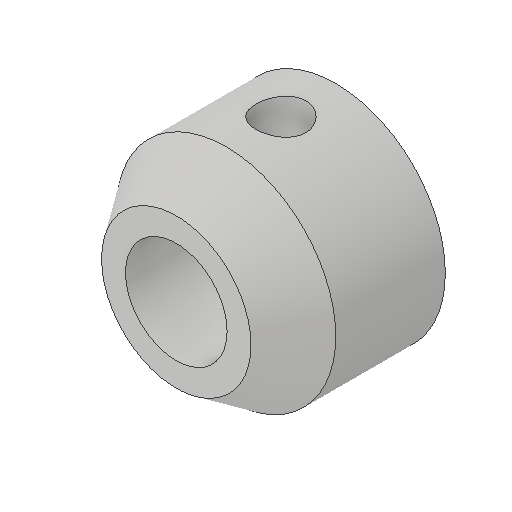
# Autodesk Inventor part: 3DP_PLA_X_axis_idler_shaft_locking_ring
Saved by Autodesk Inventor 2025 (Build 290162010, 162A)
## iProperties
Created: 2018-07-11
Part Number: 3DP_PLA_X_axis_idler_shaft_locking_ring
Material: Generic
Document SubType Name: Modeling
Designer: Andrzej
Density: 1 g/cm^3
Appearance: Default
Author: Andrzej
Autodesk Inventor part; units mm, degrees
ref_plane "YZ Plane" through (0, 0, 0) normal (1, 0, 0) x (0, 1, 0)
ref_plane "XZ Plane" through (0, 0, 0) normal (0, 1, 0) x (-1, 0, 0)
ref_plane "XY Plane" through (0, 0, 0) normal (0, 0, 1) x (1, 0, 0)
sketch "Sketch1" plane through (0, 0, 0) normal (0, 0, 1) x (1, 0, 0)
  circle A0 centre (0, 0) radius 2.55
  circle A1 centre (0, 0) radius 5.5
  dimension "d0" = 5.1
  dimension "d1" = 11
  constraints: 2 centre point, 2 coincident
  measures "d0" diameter of A0
  measures "d1" diameter of A1
extrude "Extrusion1" add sketch "Sketch1" along normal blind 8
chamfer "Chamfer1" distance 1.75 distance2 2.5 1 edges at (-5.5, 0, 8) measured on face at (-5, 0, 8)
sketch "Sketch2" plane through (0, 0, 0) normal (0, 1, 0) x (-1, 0, 0)
  line L0 (-5.5, 0) -> (5.5, 0) projected
  line L1 (5.5, 5.5) -> (-5.5, 5.5) projected
  line L2 (-5.5, 0) -> (-5.5, 5.5) projected
  line L3 (5.5, 0) -> (5.5, 5.5) projected
  point P0 (0, 0)
  point P1 (0, 2.75)
  dimension "d7" = 11
  dimension "d8" = 5.5
  dimension "d9" = 5.5
  dimension "d10" = 2.75
  measures "d7" distance of L0.start L0.end
  measures "d8" distance from line of L2 point (0, 2.75)
  measures "d9" distance between parallel lines of L0 L1
  measures "d10" distance from line of L1 point (0, 2.75)
hole "Hole1" at (0, 0, 2.75) direction (0, 1, 0) diameter 2.5 end through all both
equation "\"d8\" = 0.5 * d7"
equation "\"d10\" = 0.5 * d9"
body "Solid1"
